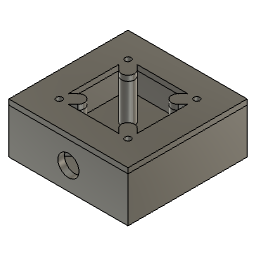
Signal_Light_Mount (Autodesk Fusion 360 design; units mm, degrees)
Autodesk Fusion 360 part; units mm, degrees
note: some values were not read from the file. Set by a fixed rule: which sketch regions a step uses.
sketch "Sketch1" plane through (0, 0, 0) normal (0, 0, 1) x (1, 0, 0)
  line L0 (0, 0) -> (90, 0)
  line L1 (90, 0) -> (90, 90)
  line L2 (90, 90) -> (0, 90)
  line L3 (0, 90) -> (0, 0)
  line L4 (10, 10) -> (80, 10) construction
  line L5 (80, 10) -> (80, 80) construction
  line L6 (80, 80) -> (10, 80) construction
  line L7 (10, 80) -> (10, 10) construction
  line L8 (45, 80) -> (45, 90) construction
  line L9 (80, 45) -> (90, 45) construction
  line L10 (19.025, 70.975) -> (70.975, 70.975) construction
  line L11 (70.975, 70.975) -> (70.975, 19.025) construction
  line L12 (70.975, 19.025) -> (19.025, 19.025) construction
  line L13 (19.025, 19.025) -> (19.025, 70.975) construction
  line L14 (45, 70.975) -> (45, 80) construction
  line L15 (70.975, 45) -> (80, 45) construction
  circle A0 centre (70.975, 70.975) radius 2.75
  circle A1 centre (70.975, 19.025) radius 2.75
  circle A2 centre (19.025, 19.025) radius 2.75
  circle A3 centre (19.025, 70.975) radius 2.75
  line L16 (26, 64) -> (64, 64) construction
  line L17 (64, 64) -> (64, 26) construction
  line L18 (64, 26) -> (26, 26) construction
  line L19 (26, 26) -> (26, 64) construction
  line L20 (45, 64) -> (45, 70.975) construction
  line L21 (64, 45) -> (70.975, 45) construction
  circle A4 centre (64, 64) radius 5
  circle A5 centre (64, 26) radius 5
  circle A6 centre (26, 26) radius 5
  circle A7 centre (26, 64) radius 5
  circle A8 centre (19.025, 70.975) radius 5
  circle A9 centre (70.975, 70.975) radius 5
  circle A10 centre (70.975, 19.025) radius 5
  circle A11 centre (19.025, 19.025) radius 5
  line L22 (60.4645, 67.5355) -> (67.4395, 74.5105)
  line L23 (74.5105, 67.4395) -> (67.5355, 60.4645)
  line L24 (67.5355, 29.5355) -> (74.5105, 22.5605)
  line L25 (60.4645, 22.4645) -> (67.4395, 15.4895)
  line L26 (22.5605, 15.4895) -> (29.5355, 22.4645)
  line L27 (22.4645, 29.5355) -> (15.4895, 22.5605)
  line L28 (22.5605, 74.5105) -> (29.5355, 67.5355)
  line L29 (15.4895, 67.4395) -> (22.4645, 60.4645)
  line L30 (5, 85) -> (85, 85)
  line L31 (85, 85) -> (85, 5)
  line L32 (85, 5) -> (5, 5)
  line L33 (5, 5) -> (5, 85)
  line L34 (45, 85) -> (45, 90) construction
  line L35 (85, 45) -> (90, 45) construction
  line L36 (18.977, 26.048) -> (18.977, 63.952)
  line L37 (26.048, 71.023) -> (63.952, 71.023)
  line L38 (71.023, 63.952) -> (71.023, 26.048)
  line L39 (63.952, 18.977) -> (26.048, 18.977)
  line L40 (3, 87) -> (87, 87)
  line L41 (87, 87) -> (87, 3)
  line L42 (87, 3) -> (3, 3)
  line L43 (3, 3) -> (3, 87)
  line L44 (2.5, 87.5) -> (87.5, 87.5)
  line L45 (87.5, 87.5) -> (87.5, 2.5)
  line L46 (87.5, 2.5) -> (2.5, 2.5)
  line L47 (2.5, 2.5) -> (2.5, 87.5)
  circle A12 centre (10, 80) radius 2.25
  circle A13 centre (80, 80) radius 2.25
  circle A14 centre (10, 10) radius 2.25
  circle A15 centre (80, 10) radius 2.25
  circle A16 centre (19.025, 70.975) radius 2.25
  circle A17 centre (70.975, 70.975) radius 2.25
  circle A18 centre (70.975, 19.025) radius 2.25
  circle A19 centre (19.025, 19.025) radius 2.25
  point P0 (45, 87)
  point P1 (45, 87.5)
  point P2 (87.5, 45)
  point P3 (87, 45)
  dimension "d1" = 70
  dimension "d2" = 90
  dimension "d3" = 51.95
  dimension "d4" = 5.5
  dimension "d5" = 10
  dimension "d6" = 38
  dimension "d7" = 10
  dimension "d8" = 5
  dimension "d19" = 2
  dimension "d20" = 0.5
  dimension "d29" = 4.5
  dimension "d31" = 4.5
  constraint horizontal L0
  constraint vertical L1
  constraint horizontal L2
  constraint vertical L3
  constraint coincident L0.start L3.end
  constraint horizontal L4
  constraint vertical L5
  constraint horizontal L6
  constraint vertical L7
  constraint midpoint L6 L8.start
  constraint midpoint L2 L8.end
  constraint midpoint L5 L9.start
  constraint midpoint L1 L9.end
  constraint vertical L8
  constraint horizontal L9
  constraint equal L5 L6
  constraint equal L0 L3
  constraint horizontal L10
  constraint vertical L11
  constraint horizontal L12
  constraint vertical L13
  constraint midpoint L10 L14.start
  constraint midpoint L11 L15.start
  constraint vertical L14
  constraint horizontal L15
  constraint equal L10 L11
  constraint coincident L10.end L11.start
  constraint coincident L11.end L12.start
  constraint coincident L12.end L13.start
  constraint coincident L10.start L13.end
  constraint equal A0 A3
  constraint equal A0 A1
  constraint equal A1 A2
  constraint horizontal L16
  constraint vertical L17
  constraint horizontal L18
  constraint vertical L19
  constraint midpoint L16 L20.start
  constraint midpoint L17 L21.start
  constraint vertical L20
  constraint horizontal L21
  constraint equal L16 L17
  constraint coincident L16.end L17.start
  constraint coincident L17.end L18.start
  constraint coincident L18.end L19.start
  constraint coincident L16.start L19.end
  constraint equal A4 A7
  constraint equal A4 A5
  constraint equal A5 A6
  constraint concentric A3 A8
  constraint concentric A0 A9
  constraint concentric A1 A10
  constraint concentric A2 A11
  constraint equal A8 A11
  constraint equal A10 A11
  constraint equal A9 A10
  constraint coincident A4 L22.start
  constraint coincident A9 L22.end
  constraint tangent A9 L22
  constraint coincident A9 L23.start
  constraint coincident A4 L23.end
  constraint tangent A4 L23
  constraint coincident A5 L24.start
  constraint coincident A10 L24.end
  constraint tangent A10 L24
  constraint coincident A5 L25.start
  constraint coincident A10 L25.end
  constraint tangent A10 L25
  constraint coincident A11 L26.start
  constraint coincident A6 L26.end
  constraint tangent A6 L26
  constraint coincident A6 L27.start
  constraint coincident A11 L27.end
  constraint tangent A11 L27
  constraint coincident A8 L28.start
  constraint parallel L25 L28
  constraint coincident A7 L28.end
  constraint tangent A7 L28
  constraint coincident A8 L29.start
  constraint coincident A7 L29.end
  constraint tangent A7 L29
  constraint tangent A8 L29
  constraint tangent A8 L28
  constraint tangent A4 L22
  constraint tangent A9 L23
  constraint tangent A5 L24
  constraint tangent A11 L26
  constraint tangent A6 L27
  constraint horizontal L30
  constraint vertical L31
  constraint horizontal L32
  constraint vertical L33
  constraint midpoint L30 L34.start
  constraint midpoint L31 L35.start
  constraint horizontal L35
  constraint vertical L34
  constraint equal L30 L31
  constraint midpoint L27 L36.start
  constraint midpoint L29 L36.end
  constraint midpoint L28 L37.start
  constraint midpoint L22 L37.end
  constraint midpoint L23 L38.start
  constraint midpoint L24 L38.end
  constraint midpoint L25 L39.start
  constraint midpoint L26 L39.end
  constraint horizontal L40
  constraint vertical L41
  constraint horizontal L42
  constraint vertical L43
  constraint horizontal L44
  constraint vertical L45
  constraint horizontal L46
  constraint vertical L47
  constraint midpoint L40 P0
  constraint midpoint L44 P1
  constraint midpoint L45 P2
  constraint midpoint L41 P3
  constraint coincident L9 P3
  constraint coincident L9 P2
  constraint coincident L34 P1
  constraint coincident L34 P0
  constraint equal L44 L45
  constraint equal L40 L41
  constraint coincident L6.end L7.start
  constraint coincident L5.end L6.start
  constraint coincident L4.start L7.end
  constraint coincident L4.end L5.start
  constraint equal A12 A13
  constraint equal A13 A15
  constraint equal A14 A15
  constraint concentric A3 A16
  constraint concentric A0 A17
  constraint concentric A10 A18
  constraint concentric A2 A19
  constraint equal A18 A19
  constraint equal A16 A18
  constraint equal A16 A17
  measures "d1" distance of L4.start L4.end
  measures "d2" distance of L0.start L0.end
  measures "d3" distance of L11.end L12.end
  measures "d4" diameter of A0
  measures "d5" diameter of A4
  measures "d6" distance of L17.end L18.end
  measures "d7" diameter of A9
  measures "d8" distance of L2 L30
  measures "d19" distance of L30 L40
  measures "d20" distance of L40 L44
  measures "d29" diameter of A12
  measures "d31" diameter of A17
extrude "Extrude1" add sketch "Sketch1" along normal blind 4 contours L0 L1 L2 L3 | A0 | A1 | A2 | A3 | A4 A9 | A4 A9 L22 | A4 A5 A6 A7 L22 L23 L24 L25 L26 L27 L28 L29 L36 L37 L38 L39 | A4 A9 L23 | A4 A9 | A4 A9 | A7 A8 L28 | A5 A10 L24 | A7 A8 | A7 A8 | A5 A10 | A5 A10 | A7 A8 L29 | A7 A8 | A5 A10 L25 | A5 A10 | A6 A11 L27 | A6 A11 L26 | A6 A11 | A6 A11 | A6 A11 | L30 L31 L32 L33 | L40 L41 L42 L43 | L44 L45 L46 L47 | A16 | A17 | A18 | A19 makes body 1
extrude "Extrude2" add sketch "Sketch1" along normal blind 34 contours L0 L1 L2 L3 | A4 A9 | A4 A9 L22 | A4 A9 L23 | A4 A9 | A4 A9 | A7 A8 L28 | A5 A10 L24 | A7 A8 | A7 A8 | A5 A10 | A5 A10 | A7 A8 L29 | A7 A8 | A5 A10 L25 | A5 A10 | A6 A11 L27 | A6 A11 L26 | A6 A11 | A6 A11 | A6 A11 | L40 L41 L42 L43 | L44 L45 L46 L47 bodies 1
extrude "Extrude3" add sketch "Sketch1" along normal blind 4 from surface at 34 separate body contours L0 L1 L2 L3 | A0 | A1 | A2 | A3 | A4 A9 | A4 A9 L22 | A4 A9 L23 | A4 A9 | A4 A9 | A7 A8 L28 | A5 A10 L24 | A7 A8 | A7 A8 | A5 A10 | A5 A10 | A7 A8 L29 | A7 A8 | A5 A10 L25 | A5 A10 | A6 A11 L27 | A6 A11 L26 | A6 A11 | A6 A11 | A6 A11 | L30 L31 L32 L33 | L40 L41 L42 L43 | L44 L45 L46 L47 | A12 | A13 | A14 | A15 makes body 2
sketch "Sketch2" plane through (0, 0, 0) normal (0, -1, 0) x (1, 0, 0)
  line L0 (0, 0) -> (90, 0)
  line L1 (90, 0) -> (90, 34)
  line L2 (90, 34) -> (0, 34)
  line L3 (0, 34) -> (0, 0)
  line L4 (45, 34) -> (45, 0) construction
  line L5 (0, 17) -> (90, 17) construction
  circle A0 centre (45, 17) radius 8
  dimension "d16" = 16
  constraint midpoint L2 L4.start
  constraint midpoint L0 L4.end
  constraint midpoint L3 L5.start
  constraint midpoint L1 L5.end
  constraint midpoint L5 A0.centre
  measures "d16" diameter of A0
extrude "Extrude4" cut sketch "Sketch2" against normal blind 9 contours A0 bodies 1
extrude "Extrude5" cut sketch "Sketch1" against normal blind 3 from surface at 34 contours L40 L41 L42 L43 | L44 L45 L46 L47 bodies 1
extrude "Extrude6" add sketch "Sketch1" against normal blind 2.8 from surface at 34 contours L40 L41 L42 L43 bodies 2
chamfer "Chamfer1" distance 1 angle 45 4 edges at (7.9023, 80.8136, 4) (77.9023, 80.8136, 4) (77.9023, 10.8136, 4) (7.9023, 10.8136, 4) on bodies 1
equation "d3 = ( ( 57.7 + 46.2 ) / 2 ) * 1 mm"
named bodies: "Signal_Lamp_Mount_bot", "Signal_Lamp_Mount_top"
